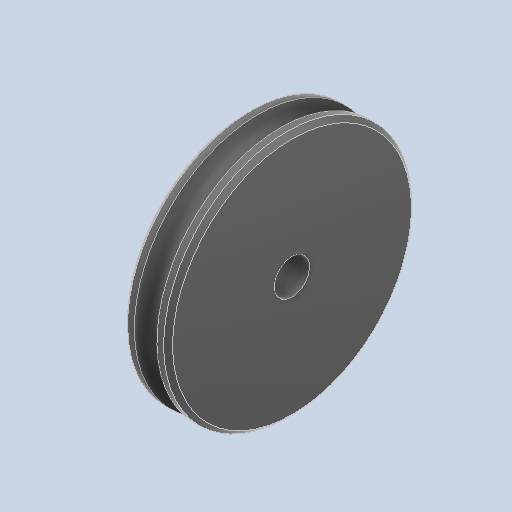
# Autodesk Inventor part: measuring_wheel_V1
Saved by Autodesk Inventor 2023 (Build 270158000, 158)
## iProperties
Created: 2023-02-13
Part Number: measuring_wheel_V1
Material: ABS-Kunststoff
Document SubType Name: Modeling
Designer: Mathi
Density: 1.06 g/cm^3
Appearance: Glatt - Weiß
Author: Mathi
Autodesk Inventor part; units mm, degrees
ref_plane "YZ Plane" through (0, 0, 0) normal (1, 0, 0) x (0, 1, 0)
ref_plane "XZ Plane" through (0, 0, 0) normal (0, 1, 0) x (-1, 0, 0)
ref_plane "XY Plane" through (0, 0, 0) normal (0, 0, 1) x (1, 0, 0)
sketch "Skizze1" plane through (0, 0, 0) normal (0, 0, 1) x (1, 0, 0)
  line L0 (-65.6518, 0) -> (54.2706, 0)
  line L1 (-11, 3.9) -> (5, 3.9)
  line L2 (4, 27.5) -> (2.5, 27.5)
  line L3 (-2.5, 27.5) -> (-4, 27.5)
  line L4 (-5, 26.5) -> (-5, 22.5)
  line L5 (-4, 21.5) -> (-3, 21.5)
  line L6 (-1, 19.5) -> (-1, 12)
  line L7 (-3, 10) -> (-10, 10)
  line L8 (-11, 9) -> (-11, 3.9)
  arc A0 (-2.5, 27.5) -> (2.5, 27.5) centre (0, 27.5) ccw
  line L9 (-4, 27.5) -> (-5, 26.5)
  line L10 (4, 27.5) -> (5, 26.5)
  line L11 (-4, 21.5) -> (-5, 22.5)
  arc A1 (-1, 19.5) -> (-3, 21.5) centre (-3, 19.5) ccw
  arc A2 (-3, 10) -> (-1, 12) centre (-3, 12) ccw
  line L12 (-10, 10) -> (-11, 9)
  line L13 (5, 26.5) -> (5, 3.9)
  line L14 (0, 27.5) -> (0, 0) construction
  point P0 (5, 27.5)
  point P1 (-5, 27.5)
  point P2 (-5, 21.5)
  point P3 (-11, 10)
  dimension "d0" = 5
  dimension "d1" = 55
  dimension "d2" = 7.8
  dimension "d3" = 20
  dimension "d6" = 6
  dimension "d8" = 1
  dimension "d9" = 1
  dimension "d10" = 1
  dimension "d11" = 1
  dimension "d12" = 1
  dimension "d13" = 1
  dimension "d14" = 2
  dimension "d15" = 1
  dimension "d16" = 1
  dimension "d19" = 6
  dimension "d20" = 10
  dimension "d21" = 6
  constraints: 30 end point, 11 point on line, 6 perpendicular, 6 point on circle, 4 tangent, 3 centre point, 1 collinear, 1 equal radius, 1 horizontal, 1 parallel, 1 vertical
  measures "d0" distance of L2.end L3.start
  measures "d1" diameter of L2 L0
  measures "d2" diameter of L1 L0
  measures "d3" diameter of L7 L0
  measures "d6" distance between parallel lines of L5 L3
  measures "d8" distance of L3.end point (-5, 27.5)
  measures "d9" distance of L4.start point (-5, 27.5)
  measures "d10" distance of L2.start point (5, 27.5)
  measures "d11" distance of L10.end point (5, 27.5)
  measures "d12" distance of L5.start point (-5, 21.5)
  measures "d13" distance of L4.end point (-5, 21.5)
  measures "d14" radius of A1
  measures "d15" distance of L7.end point (-11, 10)
  measures "d16" distance of L8.start point (-11, 10)
  measures "d19" distance between parallel lines of L13 L6
  measures "d20" distance between parallel lines of L13 L4
  measures "d21" distance between parallel lines of L4 L8
revolve "Umdrehung1" add sketch "Skizze1" angle 360 about axis through (-65.6518, 0, 0) along (1, 0, 0)
equation "\"d9\" = d8"
equation "\"d10\" = d8"
equation "\"d11\" = d10"
equation "\"d13\" = d12"
equation "\"d16\" = d15"
